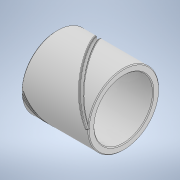
# Autodesk Inventor part: 74. Втулка распорная
Saved by Autodesk Inventor 2021 (Build 250183000, 183)
## iProperties
Created: 2021-03-28
Part Number: 74. Втулка распорная
Material: Типовые
Document SubType Name: Modeling
Designer: Данил
Density: 1 g/cm^3
Appearance: По умолчанию
Author: Данил
Autodesk Inventor part; units mm, degrees
ref_plane "YZ Plane" through (0, 0, 0) normal (1, 0, 0) x (0, 1, 0)
ref_plane "XZ Plane" through (0, 0, 0) normal (0, 1, 0) x (-1, 0, 0)
ref_plane "XY Plane" through (0, 0, 0) normal (0, 0, 1) x (1, 0, 0)
sketch "Эскиз1" plane through (0, 0, 0) normal (0, 0, 1) x (1, 0, 0)
  line L0 (-21.75, 0) -> (21.75, 0)
  line L1 (-21.25, -19) -> (21.25, -19)
  line L2 (21.75, -19.5) -> (21.75, -22.5)
  line L3 (21.25, -23) -> (-21.25, -23)
  line L4 (-21.75, -22.5) -> (-21.75, -19.5)
  line L5 (-21.25, -23) -> (-21.75, -22.5)
  line L6 (21.25, -23) -> (21.75, -22.5)
  line L7 (-21.25, -19) -> (-21.75, -19.5)
  line L8 (21.25, -19) -> (21.75, -19.5)
  point P0 (0, 0)
  point P1 (0, 0)
  point P2 (-21.75, -19)
  point P3 (21.75, -23)
  point P4 (21.75, -19)
  point P5 (-21.75, -23)
  dimension "d0" = 43.5
  dimension "d1" = 38
  dimension "d2" = 46
  dimension "d3" = 0.5
  dimension "d4" = 45
  dimension "d5" = 0.5
  dimension "d6" = 45
  dimension "d7" = 0.5
  dimension "d8" = 45
  dimension "d9" = 0.5
  dimension "d10" = 45
  constraints: 18 end point, 8 point on line, 2 horizontal, 2 parallel, 2 vertical alignment, 1 coincident, 1 midpoint, 1 perpendicular
  measures "d0" distance of L0.start L0.end
  measures "d1" diameter of L1 L0
  measures "d2" diameter of L3 L0
  measures "d3" distance of L3.end point (-21.75, -23)
  measures "d4" angle of L3 L5
  measures "d5" distance of L3.start point (21.75, -23)
  measures "d6" angle of L3 L6
  measures "d7" distance of L1.start point (-21.75, -19)
  measures "d8" angle of L1 L7
  measures "d9" distance of L1.end point (21.75, -19)
  measures "d10" angle of L1 L8
revolve "Вращение1" add sketch "Эскиз1" angle 360 about axis through (-21.75, 0, 0) along (1, 0, 0)
ref_plane "РабПлоскость1" through (21.25, 0, 23) normal (0.5113969, -0.8593446, 0) x (0.8593446, 0.5113969, 0)
sketch "Эскиз2" plane through (21.25, 0, 23) normal (0.5113969, -0.8593446, 0) x (0.8593446, 0.5113969, 0)
  arc A0 (-0.8434, -0.5373) -> (0.8434, -0.5373) centre (0, 0) ccw
  line L0 (-0.8434, -0.5373) -> (-1.1151, -0.1108)
  line L1 (0.8434, -0.5373) -> (1.1151, -0.1108)
  line L2 (1.1151, -0.1108) -> (1.6151, 0)
  line L3 (-1.1151, -0.1108) -> (-1.6151, 0)
  line L4 (-1.1151, -0.1108) -> (1.1151, -0.1108) construction
  line L5 (-1.6151, 0) -> (1.6151, 0)
  line L6 (0, 0) -> (-36.5221, 0) projected
  point P0 (-18.2611, -23)
  point P1 (0, -1)
  point P2 (0, 0)
  point P3 (0, -0.1108)
  dimension "d16" = 65
  dimension "d17" = 45
  dimension "d18" = 45
  dimension "d19" = 1
  dimension "d20" = 0.5
  constraints: 12 end point, 3 horizontal alignment, 3 point on circle, 2 coincident, 2 tangent, 2 vertical alignment, 1 centre point, 1 collinear, 1 midpoint
  measures "d16" angle of L0 L1
  measures "d17" angle of L3 L0
  measures "d18" angle of L1 L2
  measures "d19" radius of A0
  measures "d20" horizontal distance of L2.end L1.end
sketch3d "3D эскиз1"
  helix H0 starts at (-21.75, 0, -23) axis through (-21.75, 0, 0) along (1, 0, 0) pitch 86 turns 0.5 hand right
sweep "Сдвиг1" cut profiles "Эскиз2" path "3D эскиз1"
pattern_circular "Круговой массив1" count 2 over 360 about axis through (0, 0, 0) along (-1, 0, 0) of "Сдвиг1"
equation "\"d5\" = d3"
equation "\"d6\" = d4"
equation "\"d7\" = d3"
equation "\"d8\" = d4"
equation "\"d9\" = d3"
equation "\"d10\" = d4"
